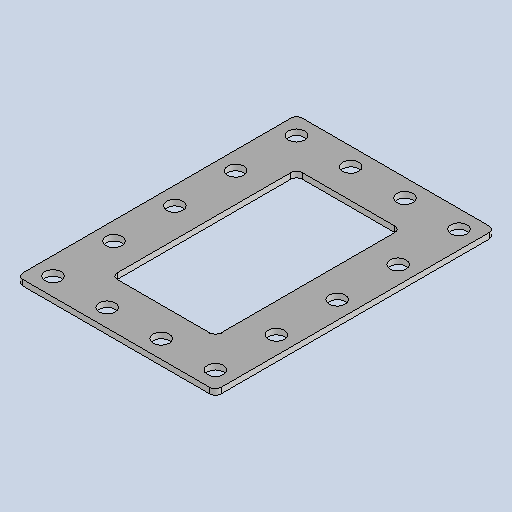
# Autodesk Inventor part: PRS 9606 charging flange round_D1200
Saved by Autodesk Inventor 2026.2 (Build 302298010, 298A)
## iProperties
Created: 2025-02-13
Part Number: PRS 9606 charging flange round_D1200
Material: Steel
Document SubType Name: Sheet Metal
Designer: admin
Mass: 2466.79 g
Surface Area: 934.137 cm^2
Volume: 314.241 cm^3
Density: 7.85 g/cm^3
Flat Pattern Width: 29.6 cm
Flat Pattern Length: 21 cm
Flat Pattern Area: 621.6 cm^2
Sheet Metal Rule: AISI304 4mm Die 32
Sheet Metal Width: 296,000 mm
Sheet Metal Length: 210,000 mm
Sheet Metal Area: 62160,000 mm^2
Appearance: Default
Author: pokla
Autodesk Inventor part; units mm, degrees
ref_plane "YZ Plane" through (0, 0, 0) normal (1, 0, 0) x (0, 1, 0)
ref_plane "XZ Plane" through (0, 0, 0) normal (0, 1, 0) x (-1, 0, 0)
ref_plane "XY Plane" through (0, 0, 0) normal (0, 0, 1) x (1, 0, 0)
sketch "Sketch2" plane through (0, 0, 0) normal (0, 0, 1) x (1, 0, 0)
  line L0 (-55, -98) -> (55, -98)
  line L1 (55, -98) -> (55, 98)
  line L2 (55, 98) -> (-55, 98)
  line L3 (-55, 98) -> (-55, -98)
  line L4 (-55, -98) -> (55, 98) construction
  line L5 (55, -98) -> (-55, 98) construction
  line L6 (-105, -148) -> (105, -148)
  line L7 (105, -148) -> (105, 148)
  line L8 (105, 148) -> (-105, 148)
  line L9 (-105, 148) -> (-105, -148)
  point P0 (0, 0)
  dimension "d29" = 110
  dimension "d30" = 196
  dimension "d31" = 50
  measures "d29" distance of L2.end L1.end
  measures "d30" distance of L1.end L0.end
  measures "d31" distance between parallel lines of L3 L9
extrude "Plate2" add sketch "Sketch2" along normal blind 6
sketch "Sketch5" plane through (0, 0, 6) normal (0, 0, 1) x (1, 0, 0)
  line L0 (55, 98) -> (55, -98) construction
  line L1 (55, -98) -> (-55, -98) construction
  line L2 (-55, -98) -> (-55, 98) construction
  line L3 (-55, 98) -> (55, 98) construction
  line L4 (105, -148) -> (-105, -148) construction
  line L5 (105, 148) -> (105, -148) construction
  line L6 (-105, 148) -> (105, 148) construction
  line L7 (-105, -148) -> (-105, 148) construction
  line L8 (-86, 129) -> (86, 129) construction
  line L9 (86, 129) -> (86, -129) construction
  line L10 (86, -129) -> (-86, -129) construction
  line L11 (-86, -129) -> (-86, 129) construction
  line L12 (-55, 0) -> (55, 0) construction
  line L13 (0, 98) -> (0, -98)
  point P0 (0, 0)
  point P1 (0, -129)
  point P2 (-86, 64.5)
  point P3 (-86, 0)
  point P4 (-86, -64.5)
  point P5 (-28.6667, -129)
  point P6 (28.6667, -129)
  point P7 (86, -64.5)
  point P8 (86, 0)
  point P9 (86, 64.5)
  point P10 (28.6667, 129)
  point P11 (-28.6667, 129)
  dimension "d34" = 19
  dimension "d49" = 64.5
  dimension "d50" = 64.5
  dimension "d51" = 57.3333
  dimension "d52" = 57.3333
  dimension "d53" = 57.3333
  constraints: 12 end point, 8 point on line, 7 midpoint, 4 coincident, 3 symmetric about line, 2 vertical alignment, 1 horizontal alignment, 3 other
  measures "d34" distance between parallel lines of L4 L10
  measures "d49" distance of point (-86, 64.5) point (-86, 129)
  measures "d50" distance of point (-86, 0) point (-86, 64.5)
  measures "d51" distance of point (-28.667, 129) point (-86, 129)
  measures "d52" distance of point (28.667, 129) point (-28.667, 129)
  measures "d53" distance of point (86, 129) point (28.667, 129)
fillet "Corner Round1" radius 6 8 edges at (-105, -148, 3) (-105, 148, 3) (105, 148, 3) (105, -148, 3) (55, -98, 3) (-55, -98, 3) (-55, 98, 3) (55, 98, 3)
hole "Hole1" at (-86, 129, 6) at (-86, 64.5, 6) at (-86, 0, 6) at (-86, -64.5, 6) at (-86, -129, 6) at (-28.6667, -129, 6) at (28.6667, -129, 6) at (86, -129, 6) at (86, -64.5, 6) at (86, 0, 6) at (86, 64.5, 6) at (86, 129, 6) at (28.6667, 129, 6) at (-28.6667, 129, 6) direction (0, 0, -1) diameter 17 end through all
equation "\"d49\" = d50"
equation "\"d51\" = d53"
equation "\"d52\" = d53"
equation "\"d29\" = ChargingHatch_hight - 2 * Thickness"
equation "\"d30\" = ChargingHatch_width - 2 * Thickness"
equation "\"d59\" = Thickness"
equation "\"d14\" = Thickness"
equation "\"BendReliefWidth\" = Thickness"
equation "\"BendReliefDepth\" = 0.5 * Thickness"
equation "\"CornerReliefSize\" = 4 * Thickness"
equation "\"MinimumRemnant\" = 2 * Thickness"
equation "\"TransitionRadius\" = BendRadius"
equation "\"JacobiRadiusSize\" = BendRadius"
equation "\"GapSize\" = Thickness"
equation "\"ChargingHatch_hight\" = 122"
equation "\"Thickness\" = 6"
equation "\"ChargingHatch_width\" = 208"
equation "\"BendRadius\" = 6"
body "Solid3"
